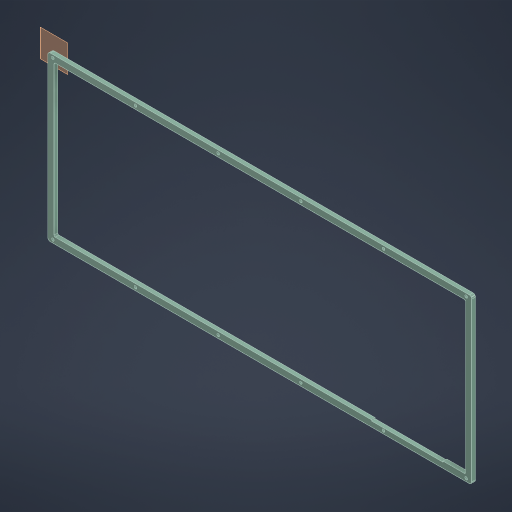
# Autodesk Inventor part: top-layer
Saved by Autodesk Inventor 2024.2 (Build 282272000, 272)
## iProperties
Created: 2024-06-20
Part Number: top-layer
Material: Generic
Document SubType Name: Modeling
Designer: Moe
Density: 1 g/cm^3
Appearance: Default
Author: Moe
Autodesk Inventor part; units mm, degrees
ref_plane "YZ Plane" through (0, 0, 0) normal (1, 0, 0) x (0, 1, 0)
ref_plane "XZ Plane" through (0, 0, 0) normal (0, 1, 0) x (-1, 0, 0)
ref_plane "XY Plane" through (0, 0, 0) normal (0, 0, 1) x (1, 0, 0)
ref_plane "Work Plane2" through (35.545, -31.609, 1.6) normal (0, 0, 1) x (1, 0, 0)
ref_plane "Work Plane1" through (35.545, -31.609, 1.6) normal (0, 0, 1) x (1, 0, 0)
sketch "Sketch1" plane through (35.545, -31.609, 1.6) normal (0, 0, 1) x (1, 0, 0)
  line L0 (0, 0) -> (336, 0) projected
  line L1 (-2, -129) -> (-2, -2) projected
  line L2 (-1.6825, -0.9187) -> (-1.5115, -0.6903) projected
  arc A0 (0, 0) -> (-2, -2) centre (0, -2) ccw
  line L3 (338, -2) -> (338, -129) projected
  line L4 (337.5115, -0.6903) -> (337.6825, -0.9187) projected
  arc A1 (338, -2) -> (336, 0) centre (336, -2) ccw
  line L5 (336, -131) -> (0, -131) projected
  line L6 (337.6825, -130.0813) -> (337.5115, -130.3097) projected
  arc A2 (336, -131) -> (338, -129) centre (336, -129) ccw
  arc A3 (-2, -129) -> (0, -131) centre (0, -129) ccw
  circle A4 centre (1.98, -128.63) radius 1.1 projected
  circle A5 centre (1.98, -128.63) radius 1.1
  circle A6 centre (68.313, -128.63) radius 1.1 projected
  circle A7 centre (134.646, -128.63) radius 1.1 projected
  circle A8 centre (134.646, -128.63) radius 1.1
  circle A9 centre (68.313, -128.63) radius 1.1
  circle A10 centre (200.979, -128.63) radius 1.1 projected
  circle A11 centre (267.312, -128.63) radius 1.1 projected
  circle A12 centre (333.645, -128.63) radius 1.1 projected
  circle A13 centre (333.645, -128.63) radius 1.1
  circle A14 centre (267.312, -128.63) radius 1.1
  circle A15 centre (200.979, -128.63) radius 1.1
  circle A16 centre (333.638, -2.355) radius 1.1 projected
  circle A17 centre (1.973, -2.355) radius 1.1 projected
  circle A18 centre (68.306, -2.355) radius 1.1 projected
  circle A19 centre (134.639, -2.355) radius 1.1 projected
  circle A20 centre (200.972, -2.355) radius 1.1 projected
  circle A21 centre (267.305, -2.355) radius 1.1 projected
  circle A22 centre (333.645, -2.355) radius 1.093
  circle A23 centre (267.305, -2.355) radius 1.1
  circle A24 centre (200.972, -2.355) radius 1.1
  circle A25 centre (134.639, -2.355) radius 1.1
  circle A26 centre (68.306, -2.355) radius 1.1
  circle A27 centre (1.973, -2.355) radius 1.1
  line L7 (3, -4.2357) -> (125.2758, -4.2357) construction
  line L8 (4, -5) -> (332, -5)
  line L9 (333, -6) -> (333, -125)
  line L10 (332, -126) -> (4, -126)
  line L11 (3, -125) -> (3, -6)
  arc A28 (4, -5) -> (3, -6) centre (4, -6) ccw
  arc A29 (333, -6) -> (332, -5) centre (332, -6) ccw
  arc A30 (332, -126) -> (333, -125) centre (332, -125) ccw
  arc A31 (3, -125) -> (4, -126) centre (4, -125) ccw
  circle A32 centre (320.737, -95.692) radius 0.175 projected
  line L12 (257.6125, -126) -> (315.0362, -126)
  line L13 (315.0362, -126) -> (315.0362, -126.7604)
  line L14 (315.0362, -126.7604) -> (257.6125, -126.7604)
  line L15 (257.6125, -126.7604) -> (257.6125, -126)
  line L16 (-4.5349, 3.2263) -> (341.5565, 3.0802) construction
  line L17 (341.5565, 3.0802) -> (341.4987, -133.8681) construction
  line L18 (341.4987, -133.8681) -> (-4.5927, -133.7221) construction
  line L19 (-4.5927, -133.7221) -> (-4.5349, 3.2263) construction
  line L20 (79.6209, -126) -> (189.9584, -126)
  line L21 (189.9584, -126) -> (189.9584, -126.7604)
  line L22 (189.9584, -126.7604) -> (79.6209, -126.7604)
  line L23 (79.6209, -126.7604) -> (79.6209, -126)
  point P0 (-35.545, 31.609)
  point P1 (-1.5115, -130.3097)
  point P2 (162.5077, 0)
  point P3 (162.5077, -5)
  point P4 (173.4174, -5)
  point P5 (173.4174, 0)
  point P6 (333, -88.192)
  point P7 (338, -88.192)
  point P8 (333, -102.192)
  point P9 (338, -102.192)
  point P10 (335.5, -88.192)
  point P11 (0, -131)
  point P12 (337.6825, -130.0813)
  point P13 (-1.6825, -0.9187)
  point P14 (337.6825, -0.9187)
  dimension "d2" = 5
  dimension "d3" = 5
  dimension "d4" = 5
  dimension "d5" = 5
  dimension "d6" = 1
  dimension "d7" = 1
  dimension "d8" = 1
  dimension "d9" = 1
  constraints: 26 end point, 20 centre point, 20 point on circle, 12 tangent, 11 coincident, 10 point on line, 6 parallel, 5 concentric, 4 horizontal, 3 perpendicular, 2 other
  measures "d2" distance between parallel lines of L3 L9
  measures "d3" distance between parallel lines of L5 L10
  measures "d4" distance between parallel lines of L1 L11
  measures "d5" distance between parallel lines of L0 L8
  measures "d6" radius of A28
  measures "d7" radius of A29
  measures "d8" radius of A30
  measures "d9" radius of A31
extrude "Extrusion3" add sketch "Sketch1" along normal blind 3 contours L0 A1 L4 L3 A2 L6 L5 A3 L1 A0 L2 | L10 L21 L22 L23
body "Solid1"
